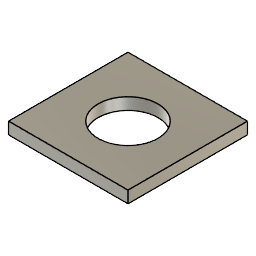
washer (Autodesk Fusion 360 design; units mm, degrees)
part number: 2025-09-15-12-59-54-930
part number: 2025-09-15-13-22-22-081
Autodesk Fusion 360 part; units mm, degrees
sketch "Sketch1" plane through (0, 0, 0) normal (0, 0, 1) x (1, 0, 0) in component "Washer"
  line L0 (100, -100) -> (-100, -100)
  line L1 (-100, -100) -> (-100, 100)
  line L2 (-100, 100) -> (100, 100)
  line L3 (100, 100) -> (100, -100)
  line L4 (100, -100) -> (-100, 100) construction
  line L5 (-100, -100) -> (100, 100) construction
  circle A0 centre (0, 0) radius 50
  dimension "d1" = 200
  dimension "d2" = 100
  constraint horizontal L0
  constraint perpendicular L0 L1
  constraint parallel L0 L2
  constraint parallel L1 L3
  constraint coincident L4 A0.centre
  constraint coincident L5 A0.centre
  constraint coincident A0.centre origin
  constraint equal L0 L1
  measures "d1" distance of L0.end L1.end
  measures "d2" diameter of A0
extrude "Extrude1" add sketch "Sketch1" along normal blind 20 in component "Washer"
component "Washer" placed x (1, 0, 0) y (0, 1, 0) z (0, 0, 1) at (0, 0, 0)
equation "d2 = d1 * 0.5"
